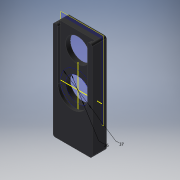
# Autodesk Inventor part: NespressoSpeedfiller
Saved by Autodesk Inventor 2017 (Build 210142000, 142)
## iProperties
Created: 2018-08-27
Part Number: NespressoSpeedfiller
Material: Generic
Document SubType Name: Modeling
Designer: 45027374
Density: 1 g/cm^3
Appearance: Default
Author: 45027374
Autodesk Inventor part; units mm, degrees
ref_plane "YZ Plane" through (0, 0, 0) normal (1, 0, 0) x (0, 1, 0)
ref_plane "XY Plane" through (0, 0, 0) normal (0, 0, 1) x (1, 0, 0)
sketch "Sketch1" plane through (0, 0, 0) normal (0, 1, 0) x (-1, 0, 0)
  line L0 (25.9, 0) -> (-25.9, 0) projected
  line L1 (0, -25.9) -> (0, 25.9) projected
  circle A0 centre (0, 0) radius 18.5 construction
  circle A1 centre (0, 0) radius 13 construction
  dimension "d0" = 37
  dimension "d1" = 26
  constraints: 2 centre point, 2 coincident
  measures "d0" diameter of A0
  measures "d1" diameter of A1
sketch "Sketch2" plane through (0, 0, 0) normal (0, 1, 0) x (-1, 0, 0)
  line L0 (29.4, 0) -> (-29.4, 0) projected
  line L1 (0, -36.3) -> (0, 70.8) projected
  line L2 (-21, 55.5) -> (-21, -21)
  line L3 (-21, -21) -> (21, -21)
  line L4 (21, -21) -> (21, 55.5)
  line L5 (-21, 55.5) -> (21, 55.5)
  point P0 (0, 0)
  dimension "d3" = 42
  dimension "d29" = 21
  dimension "d30" = 55.5
  constraints: 8 end point, 1 horizontal, 1 parallel, 1 other
  measures "d3" distance of L2.end L3.end
  measures "d29" distance between parallel lines of L0 L3
  measures "d30" distance between parallel lines of L5 L0
extrude "Extrusion1" add sketch "Sketch2" along normal blind 5
sketch "Sketch6" plane through (0, 0, 0) normal (0, 1, 0) x (-1, 0, 0)
  line L0 (21, -21) -> (-21, -21) projected
  line L1 (21, 55.5) -> (21, -21) projected
  line L2 (-21, -21) -> (21, -21)
  line L3 (21, -21) -> (21, 55.5)
  line L4 (-21, 55.5) -> (-21, -21)
  line L5 (29.4, 0) -> (-29.4, 0) projected
  line L6 (0, -36.3) -> (0, 70.8) projected
  arc A0 (-16, 0) -> (16, 0) centre (0, 0) ccw
  line L7 (16, 0) -> (16, 55.5)
  line L8 (21, 55.5) -> (-21, 55.5) projected
  line L9 (16, 55.5) -> (21, 55.5)
  line L10 (-16, 0) -> (-16, 55.5)
  line L11 (-16, 55.5) -> (-21, 55.5)
  point P0 (-17.3617, -21)
  dimension "d18" = 32
  constraints: 14 end point, 3 perpendicular, 3 point on line, 2 point on circle, 1 centre point, 1 coincident, 1 collinear, 1 horizontal, 1 parallel, 1 vertical
  measures "d18" diameter of A0
extrude "Extrusion5" add sketch "Sketch6" against normal blind 5.5 contours L0 L6 A0 L5 L1 | L0 L4 L5 A0 L6 | L5 L7 L8 L1 | L4 L8 L10 L5
sketch "Sketch4" plane through (0, 0, 0) normal (0, 0, 1) x (1, 0, 0)
  line L0 (-18.5, 0) -> (18.5, 0)
  line L1 (18.5, 0) -> (18.5, -2.5)
  line L2 (18.5, -2.5) -> (-18.5, -2.5)
  line L3 (-18.5, -2.5) -> (-18.5, 0)
  line L4 (-25.9, 0) -> (25.9, 0) projected
  line L5 (0, -2.4) -> (0, 0.4) projected
  point P0 (0, 0)
  dimension "d10" = 37
  dimension "d11" = 2.5
  constraints: 8 end point, 2 parallel, 1 collinear, 1 horizontal, 1 perpendicular, 1 other
  measures "d10" distance between parallel lines of L1 L3
  measures "d11" distance of L0.end L1.end
extrude "Extrusion6" cut sketch "Sketch4" against normal blind 21
sketch "Sketch5" plane through (0, 0, 0) normal (0, 1, 0) x (-1, 0, 0)
  circle A0 centre (0, 0) radius 18.5 construction
  circle A1 centre (0, 0) radius 18.5 construction
  line L0 (25.9, 0) -> (-25.9, 0) projected
  line L1 (0, -28.9) -> (0, 26.4) projected
  line L2 (-18.5, -21) -> (18.5, -21)
  line L3 (18.5, -21) -> (18.5, -18.5)
  line L4 (18.5, -18.5) -> (-18.5, -18.5)
  line L5 (-18.5, -18.5) -> (-18.5, -21)
  dimension "d25" = 37
  dimension "d26" = 21
  constraints: 8 end point, 2 parallel, 1 centre point, 1 coincident, 1 concentric, 1 horizontal, 1 perpendicular, 1 tangent, 1 other
  measures "d25" distance of L2.start L2.end
  measures "d26" distance between parallel lines of L0 L2
extrude "Extrusion7" add sketch "Sketch5" against normal blind 2.5
sketch "Sketch7" plane through (0, 0, 0) normal (0, 0, 1) x (1, 0, 0)
  line L0 (-18.5, 0) -> (18.5, 0)
  line L1 (18.5, 0) -> (18.5, -2.5)
  line L2 (18.5, -2.5) -> (-18.5, -2.5)
  line L3 (-18.5, -2.5) -> (-18.5, 0)
  line L4 (16, 0) -> (-16, 0) projected
  line L5 (-25.9, 0) -> (25.9, 0) projected
  line L6 (0, -2.4) -> (0, 0.4) projected
  dimension "d53" = 2.5
  dimension "d54" = 18.5
  constraints: 8 end point, 2 parallel, 1 collinear, 1 horizontal, 1 perpendicular, 1 other
  measures "d53" distance of L0.end L1.end
  measures "d54" distance between parallel lines of L6 L1
extrude "Extrusion8" cut sketch "Sketch7" along normal blind 55.5
sketch "Sketch8" plane through (0, 0, 0) normal (0, 1, 0) x (-1, 0, 0)
  circle A0 centre (0, 0) radius 13
  dimension "d34" = 26
  constraints: 1 centre point, 1 coincident
  measures "d34" diameter of A0
extrude "Extrusion9" cut sketch "Sketch8" along normal through all
pattern_linear "Rectangular Pattern1" count 2 spacing 37 along (0, 0, 1) of "Extrusion9"
sketch "Sketch9" plane through (0, 5, 0) normal (0, 1, 0) x (1, 0, 0)
  circle A0 centre (0, 0) radius 13
  circle A1 centre (0, 0) radius 15
  dimension "d40" = 26
  dimension "d41" = 30
  constraints: 2 centre point, 2 coincident
  measures "d40" diameter of A0
  measures "d41" diameter of A1
extrude "Extrusion10" [suppressed]
sketch "Sketch10" plane through (0, 5, 0) normal (0, 1, 0) x (1, 0, 0)
  arc A0 (16, 0) -> (-16, 0) centre (0, 0) ccw projected
  line L0 (1.5, -18) -> (-1.5, -18)
  line L1 (-29.4, 0) -> (29.4, 0) projected
  line L2 (0, 36.3) -> (0, -70.8) projected
  line L3 (1.5, -12) -> (-1.5, -12)
  line L4 (1.5, -12) -> (1.5, -18)
  line L5 (-1.5, -18) -> (-1.5, -12)
  dimension "d48" = 3
  dimension "d49" = 12
  dimension "d50" = 6
  constraints: 8 end point, 2 perpendicular, 1 horizontal, 1 parallel, 1 other
  measures "d48" distance between parallel lines of L4 L5
  measures "d49" distance between parallel lines of L1 L3
  measures "d50" distance between parallel lines of L0 L3
extrude "Extrusion11" [suppressed]
ref_plane "Work Plane1" through (0, 5, 0) normal (0, 1, 0) x (-1, 0, 0)
sketch "Sketch12" plane through (0, 5, 0) normal (0, 1, 0) x (-1, 0, 0)
  line L0 (21, 55.5) -> (21, -21) projected
  line L1 (21, -21) -> (-21, -21)
  line L2 (-21, -21) -> (-21, -51)
  line L3 (-21, -51) -> (21, -51)
  line L4 (21, -51) -> (21, -21)
  point P0 (0, 0)
  dimension "d61" = 42
  dimension "d62" = 30
  constraints: 8 end point, 2 parallel, 1 horizontal, 1 perpendicular
  measures "d61" distance of L2.end L3.end
  measures "d62" distance between parallel lines of L3 L1
extrude "Extrusion12" add sketch "Sketch12" against normal blind 10.5
sketch "Sketch13" plane through (0, 0, 0) normal (1, 0, 0) x (0, 1, 0)
  line L0 (-7.6, 0) -> (7.1, 0) projected
  line L1 (0, -72.3) -> (0, 76.8) projected
  line L2 (5, -51) -> (5, 55.5) projected
  line L3 (5, 55.5) -> (5, -51) projected
  line L4 (5, -49) -> (-2.5026, -49)
  line L5 (5, -49) -> (5, -21.327)
  line L6 (11.8456, -21) -> (-13.0348, -21) construction
  line L7 (5, -21) -> (-2.5026, -49)
  point P0 (0, 0)
  dimension "d70" = 49
  dimension "d71" = 21
  dimension "d72" = 15
  constraints: 8 end point, 5 point on line, 2 horizontal, 1 collinear
  measures "d70" distance between parallel lines of L0 L4
  measures "d71" distance between parallel lines of L0 L6
  measures "d72" angle of L7 L2
extrude "Extrusion14" cut sketch "Sketch13" along normal mid plane 38 contours L7 L2 L4 L1 | L1 L4 L7
fillet "Fillet2" radius 2 1 edges at (0, -2.5026, -49)
sketch "Sketch14" plane through (0, 5, 0) normal (0, 1, 0) x (-1, 0, 0)
  line L0 (19, -49) -> (-19, -49)
  line L1 (-19, -49) -> (-19, 53.5)
  line L2 (-19, 53.5) -> (19, 53.5)
  line L3 (19, 53.5) -> (19, -49)
  line L4 (21, -51) -> (-21, -51)
  line L5 (-21, -51) -> (-21, 55.5)
  line L6 (-21, 55.5) -> (21, 55.5)
  line L7 (21, 55.5) -> (21, -51)
  line L8 (-21, -51) -> (21, -51) projected
  line L9 (21, -51) -> (21, 55.5) projected
  line L10 (-21, 55.5) -> (-21, -51) projected
  line L11 (29.4, 0) -> (-29.4, 0) projected
  line L12 (0, -72.3) -> (0, 76.8) projected
  point P0 (0, 0)
  dimension "d76" = 38
  dimension "d77" = 55.5
  dimension "d78" = 53.5
  constraints: 16 end point, 4 parallel, 3 collinear, 2 horizontal, 2 perpendicular
  measures "d76" distance between parallel lines of L3 L1
  measures "d77" distance between parallel lines of L6 L11
  measures "d78" distance between parallel lines of L2 L11
extrude "Extrusion15" add sketch "Sketch14" along normal blind 5 contours L3 L11 L7 L4 L12 L0 | L12 L4 L5 L11 L1 L0 | L3 L2 L12 L6 L7 L11 | L11 L5 L6 L12 L2 L1
fillet "Fillet3" radius 2 4 edges at (21, 2.25, 55.5) (21, 2.25, -51) (-21, 2.25, -51) (-21, 2.25, 55.5)
fillet "Fillet4" radius 2 2 edges at (16, -4, 55.5) (-16, -4, 55.5)
body "Solid1"
